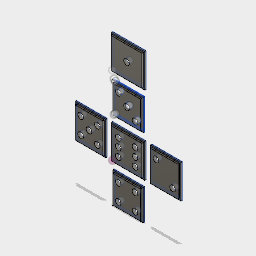
die v7 (Autodesk Fusion 360 design; units mm, degrees)
Autodesk Fusion 360 part; units mm, degrees
sketch "Sketch1" plane through (0, 0, 0) normal (0, 0, 1) x (1, 0, 0)
  line L0 (0, 0) -> (152.4, 0)
  line L1 (152.4, 0) -> (152.4, 152.4)
  line L2 (152.4, 152.4) -> (0, 152.4)
  line L3 (0, 152.4) -> (0, 0)
  circle A0 centre (38.1, 38.1) radius 12.7
  circle A1 centre (38.1, 114.3) radius 12.7
  circle A2 centre (114.3, 114.3) radius 12.7
  circle A3 centre (114.3, 38.1) radius 12.7
  circle A4 centre (114.3, 76.2) radius 12.7
  circle A5 centre (38.1, 76.2) radius 12.7
  circle A6 centre (76.2, 431.8) radius 12.7
  line L4 (152.4, 508) -> (0, 508)
  line L5 (152.4, 355.6) -> (152.4, 508)
  line L6 (0, 508) -> (0, 355.6)
  line L7 (0, 355.6) -> (152.4, 355.6)
  circle A7 centre (-95.25, 76.2) radius 12.7
  circle A8 centre (-57.15, 38.1) radius 12.7
  circle A9 centre (-57.15, 114.3) radius 12.7
  line L8 (-165.1, 0) -> (-25.4, 0)
  line L9 (-25.4, 152.4) -> (-165.1, 152.4)
  circle A10 centre (-133.35, 114.3) radius 12.7
  circle A11 centre (-133.35, 38.1) radius 12.7
  circle A12 centre (285.75, 38.1) radius 12.7
  circle A13 centre (209.55, 114.3) radius 12.7
  circle A14 centre (114.3, -63.5) radius 12.7
  circle A15 centre (38.1, -63.5) radius 12.7
  line L10 (12.7, -38.1) -> (139.7, -38.1)
  line L11 (139.7, -38.1) -> (139.7, -165.1)
  line L12 (12.7, -165.1) -> (12.7, -38.1)
  circle A16 centre (38.1, -139.7) radius 12.7
  circle A17 centre (114.3, -139.7) radius 12.7
  line L13 (139.7, -165.1) -> (12.7, -165.1)
  circle A18 centre (76.2, 254) radius 12.7
  circle A19 centre (114.3, 215.9) radius 12.7
  line L14 (139.7, 317.5) -> (139.7, 190.5)
  line L15 (139.7, 190.5) -> (12.7, 190.5)
  line L16 (12.7, 317.5) -> (139.7, 317.5)
  circle A20 centre (38.1, 292.1) radius 12.7
  line L17 (12.7, 190.5) -> (12.7, 317.5)
  line L18 (6.35, 146.05) -> (146.05, 146.05)
  line L19 (146.05, 146.05) -> (146.05, 6.35)
  line L20 (146.05, 6.35) -> (6.35, 6.35)
  line L21 (6.35, 6.35) -> (6.35, 146.05)
  line L22 (6.35, 501.65) -> (146.05, 501.65)
  line L23 (146.05, 501.65) -> (146.05, 361.95)
  line L24 (146.05, 361.95) -> (6.35, 361.95)
  line L25 (6.35, 361.95) -> (6.35, 501.65)
  line L26 (184.15, 146.05) -> (184.15, 6.35)
  line L27 (184.15, 6.35) -> (311.15, 6.35)
  line L28 (311.15, 146.05) -> (311.15, 6.35)
  line L29 (177.8, 152.4) -> (177.8, 0)
  line L30 (177.8, 152.4) -> (317.5, 152.4)
  line L31 (317.5, 152.4) -> (317.5, 0)
  line L32 (317.5, 0) -> (177.8, 0)
  line L33 (-165.1, 152.4) -> (-165.1, 0)
  line L34 (-158.75, 6.35) -> (-158.75, 146.05)
  line L35 (-158.75, 146.05) -> (-31.75, 146.05)
  line L36 (6.35, -31.75) -> (146.05, -31.75)
  line L37 (146.05, -31.75) -> (146.05, -171.45)
  line L38 (146.05, -171.45) -> (6.35, -171.45)
  line L39 (6.35, -171.45) -> (6.35, -31.75)
  line L40 (146.05, 323.85) -> (146.05, 184.15)
  line L41 (146.05, 184.15) -> (6.35, 184.15)
  line L42 (6.35, 184.15) -> (6.35, 323.85)
  line L43 (6.35, 323.85) -> (146.05, 323.85)
  line L44 (-25.4, 0) -> (-25.4, 152.4)
  line L45 (-31.75, 146.05) -> (-31.75, 6.35)
  line L46 (-31.75, 6.35) -> (-158.75, 6.35)
  line L47 (311.15, 146.05) -> (184.15, 146.05)
  line L48 (146.05, 184.15) -> (6.35, 184.15)
  line L49 (139.7, 190.5) -> (12.7, 190.5)
  circle A21 centre (76.2, 254) radius 12.7
  line L50 (139.7, 317.5) -> (139.7, 190.5)
  line L51 (146.05, 323.85) -> (146.05, 184.15)
  circle A22 centre (114.3, 215.9) radius 12.7
  circle A23 centre (38.1, 292.1) radius 12.7
  line L52 (12.7, 317.5) -> (139.7, 317.5)
  line L53 (6.35, 323.85) -> (146.05, 323.85)
  line L54 (146.05, 184.15) -> (6.35, 184.15)
  line L55 (139.7, 190.5) -> (12.7, 190.5)
  circle A24 centre (76.2, 254) radius 12.7
  line L56 (139.7, 317.5) -> (139.7, 190.5)
  line L57 (146.05, 323.85) -> (146.05, 184.15)
  circle A25 centre (114.3, 215.9) radius 12.7
  circle A26 centre (38.1, 292.1) radius 12.7
  line L58 (12.7, 317.5) -> (139.7, 317.5)
  line L59 (6.35, 323.85) -> (146.05, 323.85)
  point P0 (0, 355.6)
  dimension "d2" = 25.4
  dimension "d3" = 25.4
  dimension "d4" = 25.4
  dimension "d5" = 25.4
  dimension "d6" = 25.4
  dimension "d7" = 25.4
  dimension "d8" = 152.4
  dimension "d11" = 76.2
  dimension "d32" = 152.4
  dimension "d36" = 139.7
  dimension "d37" = 139.7
  dimension "d38" = 139.7
  dimension "d67" = 152.4
  dimension "d69" = 139.7
  dimension "d70" = 152.4
  dimension "d71" = 152.4
  measures "d2" diameter of A0
  measures "d3" diameter of A1
  measures "d4" diameter of A2
  measures "d5" diameter of A3
  measures "d6" diameter of A4
  measures "d7" diameter of A5
  measures "d8" distance of L0.start L0.end
  measures "d11" distance of A1.centre A2.centre
  measures "d32" distance of L8 L9
  measures "d36" distance of L33 L44
  measures "d37" distance of L36 L38
  measures "d38" distance of L37 L39
  measures "d67" distance of L31.end L30.end
  measures "d69" distance of L29.end L31.end
  measures "d70" distance of L4.end L4.start
  measures "d71" distance of L4.start L5.start
extrude "Extrude1" add sketch "Sketch1" along normal blind 6.35 contours L0 L1 L2 L3 | L18 L19 L20 L21 makes body 1
extrude "Extrude2" add sketch "Sketch1" along normal blind 12.7 contours L18 L19 L20 L21 bodies 1
extrude "Extrude3" add sketch "Sketch1" along normal blind 6.35 separate body contours L8 L9 L33 L44 | L34 L35 L45 L46 makes body 2
extrude "Extrude4" add sketch "Sketch1" along normal blind 12.7 contours L34 L35 L45 L46 bodies 2
extrude "Extrude5" add sketch "Sketch1" along normal blind 6.35 separate body contours L10 L11 L12 L13 | L36 L37 L38 L39 makes body 3
extrude "Extrude6" add sketch "Sketch1" along normal blind 12.7 contours L10 L11 L12 L13 bodies 3
extrude "Extrude7" add sketch "Sketch1" along normal blind 6.35 separate body contours L14 L15 L16 L17 L49 L50 L52 L55 L56 L58 | L40 L41 L42 L43 L48 L51 L53 L54 L57 L59 makes body 4
extrude "Extrude8" add sketch "Sketch1" along normal blind 12.7 contours L14 L15 L16 L17 L49 L50 L52 L55 L56 L58 bodies 4
extrude "Extrude9" add sketch "Sketch1" along normal blind 6.35 separate body contours L26 L27 L28 L47 | L29 L30 L31 L32 makes body 5
extrude "Extrude10" add sketch "Sketch1" along normal blind 12.7 contours L26 L27 L28 L47 bodies 5
extrude "Extrude11" add sketch "Sketch1" along normal blind 6.35 separate body contours L4 L5 L6 L7 | L22 L23 L24 L25 makes body 6
extrude "Extrude12" add sketch "Sketch1" along normal blind 12.7 contours L22 L23 L24 L25 bodies 6
named bodies: "Side 6", "Side 5", "Side 4", "Side 3", "Side 2", "Side 1"
